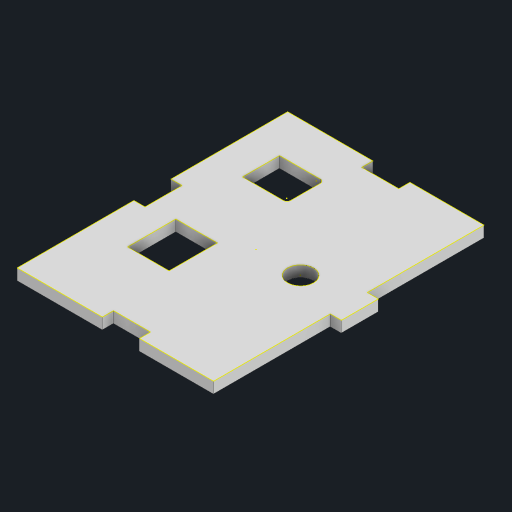
# Autodesk Inventor part: left
Saved by Autodesk Inventor 2023 (Build 270158000, 158)
## iProperties
Created: 2024-07-21
Part Number: left
Material: Generic
Document SubType Name: Modeling
Designer: Orsted
Density: 1 g/cm^3
Appearance: Default
Author: Orsted
Autodesk Inventor part; units mm, degrees
ref_plane "YZ Plane" through (0, 0, 0) normal (1, 0, 0) x (0, 1, 0)
ref_plane "XZ Plane" through (0, 0, 0) normal (0, 1, 0) x (-1, 0, 0)
ref_plane "XY Plane" through (0, 0, 0) normal (0, 0, 1) x (1, 0, 0)
sketch "Sketch1" plane through (0, 0, 0) normal (0, 1, 0) x (-1, 0, 0)
  line L0 (-28, -36.5) -> (28, -36.5)
  line L1 (28, -36.5) -> (28, 36.5)
  line L2 (28, 36.5) -> (-28, 36.5)
  line L3 (-28, 36.5) -> (-28, -36.5)
  line L4 (-28, -36.5) -> (28, 36.5) construction
  line L5 (28, -36.5) -> (-28, 36.5) construction
  point P0 (0, 0)
  dimension "d0" = 73
  dimension "d1" = 56
  constraints: 12 end point, 2 midpoint, 2 parallel, 1 horizontal, 1 perpendicular
  measures "d0" distance of L1.end L0.end
  measures "d1" distance of L0.start L0.end
extrude "Extrusion1" add sketch "Sketch1" along normal blind 3
sketch "Sketch3" plane through (0, 0, 0) normal (0, -1, 0) x (1, 0, 0)
  line L0 (-7.3, 4.62) -> (-7.3, 15.74) projected
  line L1 (-17.51, 4.16) -> (-7.86, 4.16) projected
  line L2 (-17.51, 15.74) -> (-17.51, 4.62) projected
  line L3 (-7.86, 16.2) -> (-17.51, 16.2) projected
  line L4 (-18.35, -24.665) -> (-7.85, -24.665) projected
  line L5 (-7.35, -24.165) -> (-7.35, -16.165) projected
  arc A0 (-7.85, -24.665) -> (-7.35, -24.165) centre (-7.85, -24.165) ccw projected
  arc A1 (-7.35, -16.165) -> (-7.85, -15.665) centre (-7.85, -16.165) ccw projected
  line L6 (-7.85, -15.665) -> (-18.35, -15.665) projected
  line L7 (-18.35, -15.665) -> (-18.35, -24.665)
  line L8 (-7.3, 4.62) -> (-7.3, 4.16)
  line L9 (-7.3, 4.16) -> (-7.86, 4.16)
  line L10 (-7.86, 16.2) -> (-7.3, 16.2)
  line L11 (-7.3, 16.2) -> (-7.3, 15.74)
  line L12 (-17.51, 16.2) -> (-17.51, 15.74)
  line L13 (-17.51, 4.16) -> (-17.51, 4.62)
  line L14 (-6.8, 15.74) -> (-6.8, 4.62)
  line L15 (-6.8, 4.62) -> (-6.8, 3.66)
  line L16 (-6.8, 3.66) -> (-7.86, 3.66)
  line L17 (-7.86, 3.66) -> (-18.01, 3.66)
  line L18 (-18.01, 3.66) -> (-18.01, 4.62)
  line L19 (-18.01, 4.62) -> (-18.01, 15.74)
  line L20 (-18.01, 15.74) -> (-18.01, 16.7)
  line L21 (-18.01, 16.7) -> (-7.86, 16.7)
  line L22 (-7.86, 16.7) -> (-6.8, 16.7)
  line L23 (-6.8, 16.7) -> (-6.8, 15.74)
  line L24 (-18.85, -15.165) -> (-7.85, -15.165)
  arc A2 (-6.85, -16.165) -> (-7.85, -15.165) centre (-7.85, -16.165) ccw
  line L25 (-6.85, -16.165) -> (-6.85, -24.165)
  arc A3 (-7.85, -25.165) -> (-6.85, -24.165) centre (-7.85, -24.165) ccw
  line L26 (-7.85, -25.165) -> (-18.85, -25.165)
  line L27 (-18.85, -25.165) -> (-18.85, -15.165)
  dimension "d38" = 0.5
  dimension "d39" = 0.5
  constraints: 42 end point, 6 perpendicular, 4 point on circle, 3 vertical, 2 centre point, 2 collinear, 1 point on line, 14 other
  measures "d38" distance between parallel lines of L0 L14
  measures "d39" distance between parallel lines of L6 L24
extrude "Extrusion3" cut sketch "Sketch3" against normal through all contours L8 L9 L1 L13 L2 L12 L3 L10 L11 L0 | L7 L6 A1 L5 A0 L4 | L14 L15 L16 L17 L18 L19 L20 L21 L22 L23 | L24 A2 L25 A3 L26 L27
sketch "Sketch4" plane through (0, 0, 0) normal (0, -1, 0) x (1, 0, 0)
  circle A0 centre (12, 0) radius 3.5
  line L0 (28, 36.5) -> (28, -36.5) projected
  point P0 (0, 0)
  dimension "d12" = 7
  dimension "d13" = 16
  constraints: 1 centre point
  measures "d12" diameter of A0
  measures "d13" distance from line of L0 A0.centre
extrude "Extrusion4" cut sketch "Sketch4" against normal through all
sketch "Sketch7" plane through (0, 0, 0) normal (0, -1, 0) x (1, 0, 0)
  line L0 (-5, 36.5) -> (5, 36.5)
  line L1 (5, 36.5) -> (5, 33.5)
  line L2 (5, 33.5) -> (-5, 33.5)
  line L3 (-5, 33.5) -> (-5, 36.5)
  line L4 (-5, 36.5) -> (5, 33.5) construction
  line L5 (5, 36.5) -> (-5, 33.5) construction
  line L6 (-28, 36.5) -> (28, 36.5) projected
  line L7 (-5, -36.5) -> (5, -36.5)
  line L8 (5, -36.5) -> (5, -33.5)
  line L9 (5, -33.5) -> (-5, -33.5)
  line L10 (-5, -33.5) -> (-5, -36.5)
  line L11 (-5, -36.5) -> (5, -33.5) construction
  line L12 (5, -36.5) -> (-5, -33.5) construction
  line L13 (28, -36.5) -> (-28, -36.5) projected
  line L14 (-28, -5) -> (-25, -5)
  line L15 (-25, -5) -> (-25, 5)
  line L16 (-25, 5) -> (-28, 5)
  line L17 (-28, 5) -> (-28, -5)
  line L18 (-28, -5) -> (-25, 5) construction
  line L19 (-25, -5) -> (-28, 5) construction
  line L20 (-28, -36.5) -> (-28, 36.5) projected
  line L21 (25, -5) -> (28, -5)
  line L22 (28, -5) -> (28, 5)
  line L23 (28, 5) -> (25, 5)
  line L24 (25, 5) -> (25, -5)
  line L25 (25, -5) -> (28, 5) construction
  line L26 (28, -5) -> (25, 5) construction
  line L27 (28, 36.5) -> (28, -36.5) projected
  point P0 (0, 0)
  point P1 (0, 35)
  point P2 (0, 36.5)
  point P3 (0, -35)
  point P4 (0, -36.5)
  point P5 (-26.5, 0)
  point P6 (26.5, 0)
  dimension "d26" = 10
  dimension "d27" = 3
  dimension "d28" = 10
  dimension "d29" = 3
  dimension "d30" = 3
  dimension "d31" = 10
  dimension "d32" = 3
  dimension "d33" = 10
  dimension "d36" = 36.5
  constraints: 48 end point, 12 midpoint, 8 parallel, 4 horizontal, 4 perpendicular, 1 horizontal alignment, 1 vertical alignment
  measures "d26" distance of L1.end L2.end
  measures "d27" distance of L0.end L1.end
  measures "d28" distance of L9.end L8.end
  measures "d29" distance of L8.end L7.end
  measures "d30" distance of L16.end L15.end
  measures "d31" distance of L15.end L14.end
  measures "d32" distance of L23.end L22.end
  measures "d33" distance of L22.end L21.end
  measures "d36" distance from line of point (-26.5, 0) L6
extrude "Extrusion7" cut sketch "Sketch7" against normal through all contours L0 L1 L2 L3 | L16 L15 L14 L17 | L22 L21 L24 L23 | L10 L9 L8 L7
sketch "Sketch9" plane through (0, 0, 0) normal (0, -1, 0) x (1, 0, 0)
  line L0 (25, 5) -> (28, 5) projected
  line L1 (25, 5) -> (25, 36.5)
  line L2 (5, 36.5) -> (28, 36.5) projected
  line L3 (25, -5) -> (25, 5) projected
  line L4 (25, -5) -> (25, -36.5)
  line L5 (28, -36.5) -> (5, -36.5) projected
  line L6 (28, 36.5) -> (28, 5) projected
  line L7 (28, -5) -> (25, -5) projected
  line L8 (28, 5) -> (28, -5)
  line L9 (28, -5) -> (28, -36.5) projected
  point P0 (0, 0)
  constraints: 6 end point, 3 vertical, 2 point on line
extrude "Extrusion8" add sketch "Sketch9" against normal blind 3 contours L0 L8 L7 L3
extrude "Extrusion9" cut sketch "Sketch9" against normal through all contours L1 L2 L6 L0 | L7 L9 L5 L4
sketch "Sketch10" plane through (0, 3, 0) normal (0, 1, 0) x (1, 0, 0)
  line L0 (-5, 36.5) -> (-5, 33.5) projected
  line L1 (-5, 33.5) -> (5, 33.5) projected
  line L2 (5, 33.5) -> (5, 36.5) projected
  line L3 (5, 36.5) -> (25, 36.5) projected
  line L4 (25, 36.5) -> (25, 5) projected
  line L5 (25, 5) -> (28, 5) projected
  line L6 (28, 5) -> (28, -5) projected
  line L7 (28, -5) -> (25, -5) projected
  line L8 (25, -5) -> (25, -36.5) projected
  line L9 (25, -36.5) -> (5, -36.5) projected
  line L10 (5, -36.5) -> (5, -33.5) projected
  line L11 (5, -33.5) -> (-5, -33.5) projected
  line L12 (-5, -33.5) -> (-5, -36.5) projected
  line L13 (-5, -36.5) -> (-28, -36.5) projected
  line L14 (-28, -36.5) -> (-28, -5) projected
  line L15 (-28, -5) -> (-25, -5) projected
  line L16 (-25, -5) -> (-25, 5) projected
  line L17 (-25, 5) -> (-28, 5) projected
  line L18 (-28, 5) -> (-28, 36.5) projected
  line L19 (-28, 36.5) -> (-5, 36.5) projected
  circle A0 centre (12, 0) radius 3.5 projected
  line L20 (-7.85, 25.165) -> (-18.85, 25.165) projected
  line L21 (-18.85, 25.165) -> (-18.85, 15.165) projected
  line L22 (-18.85, 15.165) -> (-7.85, 15.165) projected
  arc A1 (-7.85, 15.165) -> (-6.85, 16.165) centre (-7.85, 16.165) ccw projected
  line L23 (-6.85, 16.165) -> (-6.85, 24.165) projected
  arc A2 (-6.85, 24.165) -> (-7.85, 25.165) centre (-7.85, 24.165) ccw projected
  line L24 (-6.8, -16.7) -> (-6.8, -3.66) projected
  line L25 (-6.8, -3.66) -> (-18.01, -3.66) projected
  line L26 (-18.01, -3.66) -> (-18.01, -16.7) projected
  line L27 (-18.01, -16.7) -> (-6.8, -16.7) projected
  point P0 (0, 0)
body "Solid1"
